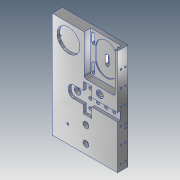
# Autodesk Inventor part: footbracket
Saved by Autodesk Inventor 2019 (Build 230136000, 136)
## iProperties
Created: 2019-01-05
Part Number: footbracket
Material: Aluminum 6061
Document SubType Name: Modeling
Designer: LillaHunden
Density: 2.7 g/cm^3
Appearance: Aluminum - Flat
Mass: 911.932 g
Surface Area: 667.083 cm^2
Volume: 337.752 cm^3
Author: LillaHunden
Autodesk Inventor part; units mm, degrees
ref_plane "YZ Plane" through (0, 0, 0) normal (1, 0, 0) x (0, 1, 0)
ref_plane "XZ Plane" through (0, 0, 0) normal (0, 1, 0) x (-1, 0, 0)
ref_plane "XY Plane" through (0, 0, 0) normal (0, 0, 1) x (1, 0, 0)
sketch "Sketch1" plane through (0, 0, 0) normal (0, 0, 1) x (1, 0, 0)
  line L0 (13.3, -8.75) -> (13.3, -10.75) construction
  line L1 (13.3, -10.75) -> (32.2, -10.75) construction
  line L2 (32.2, -10.75) -> (32.2, 3) construction
  line L3 (32.2, 3) -> (14.5, 3) construction
  line L4 (14.5, 3) -> (14.5, 0) construction
  line L5 (14.5, 0) -> (-0.1, 0) construction
  line L6 (-0.1, 0) -> (-0.1, 3) construction
  line L7 (-0.1, 3) -> (-17.8, 3) construction
  line L8 (-17.8, 3) -> (-17.8, -10.75) construction
  line L9 (-17.8, -10.75) -> (1.1, -10.75) construction
  line L10 (1.1, -10.75) -> (1.1, -8.75) construction
  line L11 (1.1, -8.75) -> (13.3, -8.75) construction
  line L12 (14.4, 0) -> (0, 0) construction
  line L13 (14.4, 0) -> (14.4, 50) construction
  line L14 (0, 50) -> (14.4, 50) construction
  line L15 (0, 0) -> (0, 50) construction
  line L16 (-60.1, -96.5) -> (59.9, -96.5)
  line L17 (59.9, -96.5) -> (59.9, 96.5)
  line L18 (59.9, 96.5) -> (-60.1, 96.5)
  line L19 (-60.1, 96.5) -> (-60.1, -96.5)
  point P0 (-60.1, 0)
  point P1 (-0.1, -96.5)
  dimension "d0" = 120
  dimension "d1" = 193
  constraints: 8 end point, 2 midpoint, 2 parallel, 1 horizontal, 1 horizontal alignment, 1 perpendicular, 1 vertical alignment
  measures "d0" distance of L18.end L17.end
  measures "d1" distance of L17.end L16.end
extrude "Extrusion1" add sketch "Sketch1" along normal mid plane 19
sketch "Sketch2" plane through (0, 0, 9.5) normal (0, 0, 1) x (1, 0, 0)
  circle A0 centre (-30.1, 68.5) radius 21
  line L0 (-60.1, 96.5) -> (-60.1, -96.5) projected
  line L1 (59.9, 96.5) -> (-60.1, 96.5) projected
  point P0 (0, 0)
  dimension "d4" = 42
  dimension "d5" = 30
  dimension "d6" = 28
  constraints: 1 centre point
  measures "d4" diameter of A0
  measures "d5" distance from line of L0 A0.centre
  measures "d6" distance from line of L1 A0.centre
extrude "Extrusion2" cut sketch "Sketch2" against normal blind 5
sketch "Sketch5" plane through (0, 0, 9.5) normal (0, 0, 1) x (1, 0, 0)
  circle A0 centre (-31.1, -64.5) radius 2
  line L0 (-60.1, -96.5) -> (59.9, -96.5) projected
  line L1 (-60.1, 96.5) -> (-60.1, -96.5) projected
  point P0 (0, 0)
  dimension "d20" = 4
  dimension "d21" = 32
  dimension "d22" = 29
  constraints: 1 centre point
  measures "d20" diameter of A0
  measures "d21" distance from line of L0 A0.centre
  measures "d22" distance from line of L1 A0.centre
extrude "Extrusion5" cut sketch "Sketch5" against normal through all
sketch "Sketch3" plane through (0, 0, 9.5) normal (0, 0, 1) x (1, 0, 0)
  circle A0 centre (1.9, -49.5) radius 5.5
  circle A1 centre (1.9, -79.5) radius 5.5
  line L0 (-60.1, 96.5) -> (-60.1, -96.5) projected
  line L1 (-60.1, -96.5) -> (59.9, -96.5) projected
  line L2 (1.9, -49.5) -> (1.9, -79.5) construction
  circle A2 centre (-31.1, -64.5) radius 2 projected
  line L3 (-31.1, -64.5) -> (-16.1488, -64.5) construction
  point P0 (0, 0)
  dimension "d9" = 11
  dimension "d10" = 11
  dimension "d11" = 62
  dimension "d25" = 47
  constraints: 4 end point, 2 centre point, 1 horizontal, 1 symmetric about line, 1 vertical, 1 vertical alignment
  measures "d9" diameter of A0
  measures "d10" diameter of A1
  measures "d11" distance from line of L0 L2.start
  measures "d25" distance from line of L1 L2.start
extrude "Extrusion3" cut sketch "Sketch3" against normal blind 7.14 contours A0 | A1
sketch "Sketch4" plane through (1.9, -49.5, 2.36) normal (0, 0, 1) x (1, 0, 0)
  circle A0 centre (0, -30) radius 5.5 projected
  circle A1 centre (0, 0) radius 5.5 projected
  circle A2 centre (0, 0) radius 3.465
  circle A3 centre (0, -30) radius 3.465
  point P0 (-1.9, 49.5)
  dimension "d16" = 6.93
  dimension "d17" = 6.93
  constraints: 2 centre point, 2 coincident
  measures "d16" diameter of A2
  measures "d17" diameter of A3
extrude "Extrusion4" cut sketch "Sketch4" against normal through all contours A2 | A3
sketch "Sketch6" plane through (0, 0, -9.5) normal (0, 0, -1) x (-1, 0, 0)
  circle A0 centre (31.1, -64.5) radius 2 projected
  circle A1 centre (31.1, -64.5) radius 21
  point P0 (0, 0)
  dimension "d26" = 42
  constraints: 1 centre point, 1 coincident
  measures "d26" diameter of A1
extrude "Extrusion6" cut sketch "Sketch6" against normal blind 5
sketch "Sketch7" plane through (0, 0, -9.5) normal (0, 0, -1) x (-1, 0, 0)
  line L0 (16.4, -52) -> (16.4, -96.5)
  line L1 (60.1, -96.5) -> (60.1, 96.5) projected
  line L2 (16.4, -52) -> (60.1, -52)
  line L3 (-59.9, -96.5) -> (60.1, -96.5) projected
  point P0 (0, 0)
  dimension "d29" = 43.7
  dimension "d30" = 44.5
  constraints: 4 end point, 2 point on line, 1 horizontal, 1 vertical
  measures "d29" distance between parallel lines of L1 L0
  measures "d30" distance between parallel lines of L3 L2
extrude "Extrusion7" cut sketch "Sketch7" against normal blind 3.3
sketch "Sketch8" plane through (0, 0, 9.5) normal (0, 0, 1) x (1, 0, 0)
  line L0 (8.9, -15.7) -> (58.9, -15.7) construction
  line L1 (58.9, -15.7) -> (58.9, -1.3) construction
  line L2 (8.9, -1.3) -> (58.9, -1.3) construction
  line L3 (-1.85, 16.5) -> (11.9, 16.5) construction
  line L4 (11.9, 16.5) -> (11.9, -1.2) construction
  line L5 (-1.85, -2.4) -> (-1.85, 16.5) construction
  line L6 (-7.85, -3) -> (-7.85, -14) construction
  line L7 (-1.85, -33.5) -> (-1.85, -14.6) construction
  line L8 (11.9, -33.5) -> (-1.85, -33.5) construction
  line L9 (11.9, -15.8) -> (11.9, -33.5) construction
  line L10 (-7.85, -3) -> (-7.85, -1) construction
  line L11 (-7.85, -1) -> (-1.85, -1) construction
  line L12 (-7.85, -14) -> (-7.85, -16) construction
  line L13 (-7.85, -16) -> (-1.85, -16) construction
  line L14 (59.9, -0.8) -> (59.9, -16.2)
  line L15 (59.9, -16.2) -> (12.4, -16.2)
  line L16 (12.4, -0.8) -> (12.4, -34)
  line L17 (12.4, -34) -> (-2.35, -34)
  line L18 (-2.35, -34) -> (-2.35, -16.5)
  line L19 (12.4, -16.2) -> (12.4, 17)
  line L20 (12.4, 17) -> (-2.35, 17)
  line L21 (-2.35, 17) -> (-2.35, -0.5)
  line L22 (-2.35, -0.5) -> (-8.35, -0.5)
  line L23 (-8.35, -0.5) -> (-8.35, -3)
  line L24 (-8.35, -3) -> (-8.35, -14)
  line L25 (-8.35, -14) -> (-8.35, -16.5)
  line L26 (-8.35, -16.5) -> (-2.35, -16.5)
  line L27 (12.4, -0.8) -> (59.9, -0.8)
  line L28 (12.4, -0.8) -> (59.9, -0.8)
  line L29 (59.9, -0.8) -> (59.9, -16.2)
  line L30 (59.9, -16.2) -> (12.4, -16.2)
  line L31 (12.4, -16.2) -> (12.4, -0.8)
  point P0 (0, 0)
  point P1 (59.9, -8.5)
  point P2 (59.9, 96.5)
  dimension "d33" = 2
  dimension "d34" = 2
  dimension "d36" = 0.5
  dimension "d38" = 0.5
  dimension "d44" = 0.5
  dimension "d45" = 0.5
  dimension "d46" = 0.5
  constraints: 44 end point, 5 point on line, 4 perpendicular, 2 parallel, 1 horizontal, 1 midpoint, 1 vertical, 1 vertical alignment, 2 other
  measures "d33" distance of L6.start L10.end
  measures "d34" distance of L6.end L12.end
  measures "d36" distance between parallel lines of L9 L16
  measures "d38" distance between parallel lines of L11 L22
  measures "d44" distance between parallel lines of L15 L0
  measures "d45" distance between parallel lines of L2 L27
  measures "d46" distance between parallel lines of L3 L20
extrude "Extrusion8" cut sketch "Sketch8" against normal blind 5 contours L16 L17 L18 L26 L25 L24 L23 L22 L21 L20 L19
sketch "Sketch9" plane through (0, 0, 9.5) normal (0, 0, 1) x (1, 0, 0)
  line L0 (-12.85, 11.5) -> (-12.85, -28.5) construction
  line L1 (-12.85, -28.5) -> (-20.85, -28.5) construction
  line L2 (-20.85, 11.5) -> (-20.85, -28.5) construction
  line L3 (-12.85, 11.5) -> (-20.85, 11.5) construction
  line L4 (-12.85, -8.5) -> (-20.85, -8.5) construction
  circle A0 centre (-18.35, -8.5) radius 6.1
  line L5 (-8.35, -16.5) -> (-8.35, -0.5) projected
  point P0 (0, 0)
  dimension "d41" = 12.2
  dimension "d116" = 10
  constraints: 2 end point, 2 midpoint, 1 centre point, 1 perpendicular, 1 point on line
  measures "d41" diameter of A0
  measures "d116" distance from line of A0.centre L5
extrude "Extrusion9" cut sketch "Sketch9" against normal through all
sketch "Sketch10" plane through (0, 0, 9.5) normal (0, 0, 1) x (1, 0, 0)
  line L0 (8.9, -15.7) -> (58.9, -15.7) construction
  line L1 (8.9, -1.3) -> (58.9, -1.3) construction
  line L2 (12.4, 17) -> (12.4, -34) construction
  line L3 (12.4, 17) -> (12.4, -34) projected
  line L4 (59.9, 96.5) -> (59.9, -96.5) projected
  line L5 (59.9, -1) -> (59.9, -16)
  line L6 (59.9, -16) -> (12.4, -16)
  line L7 (12.4, -16) -> (12.4, -1.3)
  line L8 (8.9, -1) -> (59.9, -1)
  line L9 (59.9, -96.5) -> (59.9, 96.5) projected
  line L10 (12.4, -1.3) -> (12.4, -1)
  point P0 (0, 0)
  dimension "d49" = 0.3
  dimension "d50" = 0.3
  constraints: 10 end point, 6 point on line, 2 parallel
  measures "d49" distance between parallel lines of L0 L6
  measures "d50" distance between parallel lines of L1 L8
extrude "Extrusion10" cut sketch "Sketch10" against normal up to surface (5 mm away)
sketch "Sketch12" plane through (0, 0, 9.5) normal (0, 0, 1) x (1, 0, 0)
  line L0 (55.1541, 83.9537) -> (55.1541, 33.9537) construction
  arc A0 (52.1541, 30.9537) -> (55.1541, 33.9537) centre (52.1541, 33.9537) ccw construction
  line L1 (52.1541, 30.9537) -> (2.1541, 30.9537) construction
  arc A1 (55.1541, 83.9537) -> (52.1541, 86.9537) centre (52.1541, 83.9537) ccw construction
  line L2 (2.1541, 86.9537) -> (52.1541, 86.9537) construction
  arc A2 (2.1541, 86.9537) -> (-0.8459, 83.9537) centre (2.1541, 83.9537) ccw construction
  line L3 (-0.8459, 33.9537) -> (-0.8459, 83.9537) construction
  arc A3 (-0.8459, 33.9537) -> (2.1541, 30.9537) centre (2.1541, 33.9537) ccw construction
  line L4 (-1.3459, 22.9537) -> (55.6541, 22.9537)
  line L5 (55.6541, 22.9537) -> (55.6541, 96.9537)
  line L6 (55.6541, 96.9537) -> (-1.3459, 96.9537)
  line L7 (-1.3459, 96.9537) -> (-1.3459, 22.9537)
  point P0 (0, 0)
  dimension "d54" = 8
  dimension "d55" = 0.5
  dimension "d56" = 0.5
  dimension "d57" = 10
  constraints: 8 end point, 2 parallel, 1 horizontal, 1 perpendicular, 1 other
  measures "d54" distance between parallel lines of L4 L1
  measures "d55" distance between parallel lines of L3 L7
  measures "d56" distance between parallel lines of L5 L0
  measures "d57" distance between parallel lines of L2 L6
extrude "Extrusion12" cut sketch "Sketch12" against normal blind 12
sketch "Sketch13" plane through (0, 0, -2.5) normal (0, 0, 1) x (1, 0, 0)
  circle A0 centre (50.7241, 27.8837) radius 2.6 construction
  circle A1 centre (50.7241, 75.0237) radius 2.6 construction
  circle A2 centre (3.5841, 75.0237) radius 2.6 construction
  circle A3 centre (3.5841, 27.8837) radius 2.6 construction
  line L0 (3.5841, 25.2837) -> (3.5841, 45.2837) construction
  line L1 (0.9841, 27.8837) -> (0.9841, 42.6837)
  line L2 (6.1841, 42.6837) -> (6.1841, 27.8837)
  arc A4 (0.9841, 27.8837) -> (6.1841, 27.8837) centre (3.5841, 27.8837) ccw
  arc A5 (6.1841, 42.6837) -> (0.9841, 42.6837) centre (3.5841, 42.6837) ccw
  line L3 (3.5841, 72.4237) -> (3.5841, 92.4237) construction
  line L4 (0.9841, 75.0237) -> (0.9841, 89.8237)
  line L5 (6.1841, 89.8237) -> (6.1841, 75.0237)
  arc A6 (0.9841, 75.0237) -> (6.1841, 75.0237) centre (3.5841, 75.0237) ccw
  arc A7 (6.1841, 89.8237) -> (0.9841, 89.8237) centre (3.5841, 89.8237) ccw
  line L6 (50.7241, 72.4237) -> (50.7241, 92.4237) construction
  line L7 (48.1241, 75.0237) -> (48.1241, 89.8237)
  line L8 (53.3241, 89.8237) -> (53.3241, 75.0237)
  arc A8 (48.1241, 75.0237) -> (53.3241, 75.0237) centre (50.7241, 75.0237) ccw
  arc A9 (53.3241, 89.8237) -> (48.1241, 89.8237) centre (50.7241, 89.8237) ccw
  line L9 (50.7241, 25.2837) -> (50.7241, 45.2837) construction
  line L10 (48.1241, 27.8837) -> (48.1241, 42.6837)
  line L11 (53.3241, 42.6837) -> (53.3241, 27.8837)
  arc A10 (48.1241, 27.8837) -> (53.3241, 27.8837) centre (50.7241, 27.8837) ccw
  arc A11 (53.3241, 42.6837) -> (48.1241, 42.6837) centre (50.7241, 42.6837) ccw
  point P0 (0, 0)
  point P1 (3.5841, 35.2837)
  point P2 (3.5841, 82.4237)
  point P3 (50.7241, 82.4237)
  point P4 (50.7241, 35.2837)
  dimension "d60" = 20
  dimension "d61" = 20
  dimension "d62" = 20
  dimension "d63" = 20
  dimension "d117" = 5.2
  dimension "d118" = 5.2
  constraints: 32 end point, 24 point on circle, 16 tangent, 12 point on line, 8 centre point, 5 parallel, 4 midpoint, 4 vertical alignment, 1 vertical, 4 other
  measures "d60" distance of L0.start L0.end
  measures "d61" distance of L3.start L3.end
  measures "d62" distance of L6.start L6.end
  measures "d63" distance of L9.start L9.end
  measures "d117" distance between parallel lines of L5 L4
  measures "d118" distance between parallel lines of L1 L2
extrude "Extrusion13" cut sketch "Sketch13" against normal through all
sketch "Sketch14" plane through (0, 0, -2.5) normal (0, 0, 1) x (1, 0, 0)
  circle A0 centre (27.1541, 51.4537) radius 19.5 construction
  arc A1 (7.6604, 46.9821) -> (46.6279, 46.8964) centre (27.1541, 51.4537) ccw
  line L0 (46.6279, 72.4633) -> (46.6279, 46.8964)
  line L1 (7.6604, 46.9821) -> (7.6604, 70.9586)
  arc A2 (46.6279, 70.4442) -> (7.6604, 70.9586) centre (27.1541, 71.4537) ccw
  point P0 (0, 0)
  point P1 (46.6279, 67.5038)
  point P2 (27.1541, 90.9537)
  dimension "d67" = 39
  dimension "d68" = 0.5
  dimension "d120" = 39
  dimension "d121" = 20
  constraints: 5 point on circle, 4 end point, 2 centre point, 2 point on line, 2 vertical, 2 vertical alignment
  measures "d67" diameter of A0
  measures "d68" radial gap between concentric circles of A0 A1
  measures "d120" diameter of A2
  measures "d121" distance of A0.centre A2.centre
extrude "Extrusion14" cut sketch "Sketch14" against normal blind 1.85 contours L1 A2 L0 A1
sketch "Sketch15" plane through (0, 0, -4.35) normal (0, 0, 1) x (1, 0, 0)
  circle A0 centre (27.1541, 51.4537) radius 3.18 construction
  line L0 (27.1541, 48.2737) -> (27.1541, 68.2737) construction
  line L1 (30.4041, 51.5237) -> (30.4041, 65.0237)
  line L2 (23.9041, 65.0237) -> (23.9041, 51.5237)
  arc A1 (23.9041, 51.5237) -> (30.4041, 51.5237) centre (27.1541, 51.5237) ccw
  arc A2 (30.4041, 65.0237) -> (23.9041, 65.0237) centre (27.1541, 65.0237) ccw
  point P0 (0, 0)
  point P1 (27.1541, 58.2737)
  dimension "d72" = 20
  dimension "d73" = 6.5
  constraints: 8 end point, 6 point on circle, 4 tangent, 2 centre point, 2 point on line, 1 midpoint, 1 parallel, 1 vertical, 1 vertical alignment, 1 other
  measures "d72" distance of L0.start L0.end
  measures "d73" diameter of A2
extrude "Extrusion15" cut sketch "Sketch15" against normal through all
sketch "Sketch16" plane through (0, 0, 9.5) normal (0, 0, 1) x (1, 0, 0)
  circle A0 centre (27.1817, 11.6) radius 4.7625 projected
  point P0 (0, 0)
extrude "Extrusion16" cut sketch "Sketch16" against normal through all
sketch "Sketch17" plane through (0, 0, -9.5) normal (0, 0, -1) x (-1, 0, 0)
  circle A0 centre (-48.9, -8.5) radius 2.067 construction
  circle A1 centre (-33.9, -8.5) radius 2.067 construction
  circle A2 centre (-18.9, -8.5) radius 2.067 construction
  circle A3 centre (-5.025, -24.65) radius 2.067 construction
  circle A4 centre (-5.025, -8.5) radius 2.067 construction
  circle A5 centre (-5.025, 7.65) radius 2.067 construction
  circle A6 centre (-5.025, -24.65) radius 3
  circle A7 centre (-5.025, -8.5) radius 3
  circle A8 centre (-18.9, -8.5) radius 3
  circle A9 centre (-33.9, -8.5) radius 3
  circle A10 centre (-48.9, -8.5) radius 3
  circle A11 centre (-5.025, 7.65) radius 3
  point P0 (0, 0)
  dimension "d78" = 6
  dimension "d79" = 6
  dimension "d80" = 6
  dimension "d81" = 6
  dimension "d82" = 6
  dimension "d83" = 6
  constraints: 6 centre point
  measures "d78" diameter of A7
  measures "d79" diameter of A6
  measures "d80" diameter of A11
  measures "d81" diameter of A8
  measures "d82" diameter of A9
  measures "d83" diameter of A10
extrude "Extrusion17" cut sketch "Sketch17" against normal through all
sketch "Sketch18" plane through (0, 0, -9.5) normal (0, 0, -1) x (-1, 0, 0)
  line L0 (-59.9, -1) -> (-12.4, -1) projected
  line L1 (-56.4, -8.5) -> (2.475, -8.5) construction
  line L2 (-48.9, -16) -> (-5.025, -16)
  line L3 (-5.025, -1) -> (-48.9, -1)
  arc A0 (-48.9, -1) -> (-48.9, -16) centre (-48.9, -8.5) ccw
  arc A1 (-5.025, -16) -> (-5.025, -1) centre (-5.025, -8.5) ccw
  line L4 (-5.025, -32.15) -> (-5.025, 13.5608) construction
  line L5 (-12.525, -24.65) -> (-12.525, 6.0608)
  line L6 (2.475, 6.0608) -> (2.475, -24.65)
  arc A2 (-12.525, -24.65) -> (2.475, -24.65) centre (-5.025, -24.65) ccw
  arc A3 (2.475, 6.0608) -> (-12.525, 6.0608) centre (-5.025, 6.0608) ccw
  point P0 (-5.025, 7.65)
  point P1 (-26.9625, -8.5)
  point P2 (-5.025, -9.2946)
  dimension "d94" = 7.5
  dimension "d95" = 7.5
  constraints: 16 end point, 12 point on circle, 8 tangent, 6 point on line, 4 centre point, 3 coincident, 2 midpoint, 2 parallel, 1 horizontal, 1 perpendicular
  measures "d94" radius of A2
  measures "d95" radius of A1
extrude "Extrusion18" cut sketch "Sketch18" against normal blind 7
sketch "Sketch19" plane through (0, 0, -9.5) normal (0, 0, -1) x (-1, 0, 0)
  circle A0 centre (18.35, -8.5) radius 6.1 projected
  circle A1 centre (18.35, -8.5) radius 11.7114
  point P0 (0, 0)
  constraints: 1 centre point, 1 coincident
extrude "Extrusion19" cut sketch "Sketch19" against normal up to surface (7 mm away)
fillet "Fillet1" radius 4 2 edges at (55.6541, 22.9537, 3.5) (-1.3459, 22.9537, 3.5)
sketch "Sketch20" plane through (0, 0, 9.5) normal (0, 0, 1) x (1, 0, 0)
  circle A0 centre (-18.35, -8.5) radius 6.1 projected
  arc A1 (-18.35, -0.5) -> (-18.35, -16.5) centre (-18.35, -8.5) ccw
  line L0 (-8.35, -0.5) -> (-2.35, -0.5) projected
  line L1 (-2.35, -16.5) -> (-8.35, -16.5) projected
  line L2 (-8.35, -16.5) -> (-18.35, -16.5)
  line L3 (-8.35, -0.5) -> (-18.35, -0.5)
  line L4 (-8.35, -16.5) -> (-8.35, -0.5) projected
  line L5 (-2.35, -0.5) -> (-2.35, 17) projected
  line L6 (-29.85, -19.5) -> (-2.35, -19.5)
  line L7 (-2.35, -19.5) -> (-2.35, 2.5)
  line L8 (-2.35, 2.5) -> (-29.85, 2.5)
  line L9 (-29.85, 2.5) -> (-29.85, -19.5)
  point P0 (0, 0)
  dimension "d112" = 3
  dimension "d113" = 3
  dimension "d114" = 11.5
  constraints: 12 end point, 3 parallel, 2 point on circle, 1 centre point, 1 coincident, 1 collinear, 1 horizontal, 1 perpendicular, 1 point on line, 1 tangent
  measures "d112" distance between parallel lines of L6 L1
  measures "d113" distance between parallel lines of L0 L8
  measures "d114" distance from line of L9 A1.centre
extrude "Extrusion20" cut sketch "Sketch20" against normal up to surface (5 mm away)
sketch "Sketch21" plane through (0, 0, 9.5) normal (0, 0, 1) x (1, 0, 0)
  circle A0 centre (-0.9358, -32.5858) radius 2
  line L0 (12.4, -34) -> (-2.35, -34) projected
  line L1 (-2.35, -34) -> (3.6865, -27.9635) construction
  line L2 (12.4, -16) -> (12.4, -34) projected
  line L3 (12.4, -34) -> (9.5716, -31.1716) construction
  line L4 (-2.35, 2.5) -> (-2.35, 17) projected
  line L5 (-2.35, 17) -> (2.4494, 12.2006) construction
  line L6 (12.4, 17) -> (9.5716, 14.1716) construction
  line L7 (12.4, 17) -> (12.4, -1) projected
  circle A1 centre (10.9858, -32.5858) radius 2
  circle A2 centre (-0.9358, 15.5858) radius 2
  circle A3 centre (10.9858, 15.5858) radius 2
  point P0 (0, 0)
  point P1 (-2.35, -0.5)
  dimension "d102" = 4
  dimension "d107" = 4
  dimension "d108" = 4
  dimension "d109" = 4
  dimension "d103" = 45
  dimension "d104" = 45
  dimension "d105" = 45
  dimension "d106" = 45
  constraints: 8 end point, 2 midpoint, 2 point on line, 12 other
  measures "d103" angle of L0 L1
  measures "d104" angle of L4 L5
  measures "d105" angle of L7 L6
  measures "d106" angle of L0 L3
extrude "Extrusion21" cut sketch "Sketch21" against normal up to surface (5 mm away)
fillet "Fillet2" radius 8 2 edges at (-29.85, -19.5, 7) (-29.85, 2.5, 7)
sketch "Sketch22" plane through (0, 0, 9.5) normal (0, 0, 1) x (1, 0, 0)
  circle A0 centre (27.1817, 11.6) radius 4.7625 projected
  circle A1 centre (27.1817, 11.6) radius 6.5
  point P0 (0, 0)
  dimension "d122" = 13
  constraints: 1 centre point, 1 coincident
  measures "d122" diameter of A1
extrude "Extrusion22" cut sketch "Sketch22" against normal blind 2 contours A0 | A1
sketch "Sketch23" plane through (0, 0, -9.5) normal (0, 0, -1) x (-1, 0, 0)
  circle A0 centre (-27.1817, 11.6) radius 6.5 projected
  point P0 (0, 0)
extrude "Extrusion23" cut sketch "Sketch23" against normal blind 2
sketch "Sketch24" plane through (-60.1, -96.5, 9.5) normal (-1, 0, 0) x (0, 0, 1)
  circle A0 centre (-6.3333, 160.8333) radius 2.25 construction
  circle A1 centre (-14.3333, 160.8333) radius 2.25 construction
  circle A2 centre (-14.3333, 128.6667) radius 2.25 construction
  circle A3 centre (-6.3333, 128.6667) radius 2.25 construction
  circle A4 centre (-6.3333, 96.5) radius 2.25 construction
  circle A5 centre (-14.3333, 96.5) radius 2.25 construction
  circle A6 centre (-14.3333, 64.3333) radius 2.25 construction
  circle A7 centre (-6.3333, 64.3333) radius 2.25 construction
  circle A8 centre (-6.3333, 32.1667) radius 2.25 construction
  circle A9 centre (-14.3333, 32.1667) radius 2.25 construction
  point P0 (-9.5, 96.5)
  constraints: 1 centre point
hole "Hole1" at (-60.1, 64.3333, -4.8333) at (-60.1, 64.3333, 3.1667) at (-60.1, 32.1667, 3.1667) at (-60.1, 32.1667, -4.8333) at (-60.1, 0, -4.8333) at (-60.1, 0, 3.1667) at (-60.1, -32.1667, 3.1667) at (-60.1, -32.1667, -4.8333) at (-60.1, -64.3333, 3.1667) direction (1, 0, 0) diameter 3.242 depth 11.8 thread size "M4x0.7" class "6H" standard "ISO Metric profile"
sketch "Sketch25" plane through (59.9, -96.5, -9.5) normal (1, 0, 0) x (0, 0, -1)
  circle A0 centre (-4.6667, 64.3333) radius 1.621 construction
  circle A1 centre (-12.6667, 96.5) radius 1.621 construction
  circle A2 centre (-4.6667, 128.6667) radius 1.621 construction
  circle A3 centre (-12.6667, 160.8333) radius 1.621 construction
  circle A4 centre (-4.6667, 160.8333) radius 1.621 construction
  circle A5 centre (-12.6667, 128.6667) radius 1.621 construction
  circle A6 centre (-4.6667, 96.5) radius 1.621 construction
  circle A7 centre (-12.6667, 64.3333) radius 1.621 construction
  circle A8 centre (-12.6667, 32.1667) radius 1.621 construction
  line L0 (0, 44.5) -> (-3.3, 44.5) construction
  line L1 (-3.3, 44.5) -> (-3.3, 0) construction
  line L2 (-19, 0) -> (-3.3, 0) construction
  line L3 (-19, 193) -> (-19, 0) construction
  line L4 (0, 193) -> (-19, 193) construction
  line L5 (0, 44.5) -> (0, 193) construction
  circle A9 centre (-4.6667, 10.8333) radius 3.25 projected
  circle A10 centre (-4.6667, 40.8333) radius 3.25 projected
  circle A11 centre (-12.6667, 70.8333) radius 3.25 projected
  circle A12 centre (-4.6667, 100.8333) radius 3.25 projected
  circle A13 centre (-4.6667, 130.8333) radius 3.25 projected
  circle A14 centre (-12.6667, 160.8333) radius 3.25 projected
  circle A15 centre (-4.6667, 160.8333) radius 3.25 projected
  circle A16 centre (-12.6667, 130.8333) radius 3.25 projected
  circle A17 centre (-12.6667, 100.8333) radius 3.25 projected
  circle A18 centre (-4.6667, 70.8333) radius 3.25 projected
  circle A19 centre (-12.6667, 40.8333) radius 3.25 projected
  circle A20 centre (-12.6667, 10.8333) radius 3.25 projected
  circle A21 centre (-22.7521, 16) radius 3.25 projected
  circle A22 centre (-22.7521, -174) radius 3.25 projected
  circle A23 centre (-22.7521, -157) radius 3.25 projected
  circle A24 centre (-22.7521, 33) radius 3.25 projected
  line L6 (4, -32.5) -> (20, -32.5) projected
  arc A25 (20, -39.5) -> (20, -32.5) centre (20, -36) ccw projected
  line L7 (20, -39.5) -> (4, -39.5) projected
  arc A26 (4, -32.5) -> (4, -39.5) centre (4, -36) ccw projected
  arc A27 (43.57, -15.03) -> (43.57, -9.83) centre (43.57, -12.43) ccw projected
  line L8 (43.57, -15.03) -> (27.57, -15.03) projected
  arc A28 (27.57, -9.83) -> (27.57, -15.03) centre (27.57, -12.43) ccw projected
  line L9 (27.57, -9.83) -> (43.57, -9.83) projected
  arc A29 (-3.57, -15.03) -> (-3.57, -9.83) centre (-3.57, -12.43) ccw projected
  line L10 (-3.57, -15.03) -> (-19.57, -15.03) projected
  arc A30 (-19.57, -9.83) -> (-19.57, -15.03) centre (-19.57, -12.43) ccw projected
  line L11 (-19.57, -9.83) -> (-3.57, -9.83) projected
  arc A31 (-3.57, -62.17) -> (-3.57, -56.97) centre (-3.57, -59.57) ccw projected
  line L12 (-3.57, -62.17) -> (-19.57, -62.17) projected
  arc A32 (-19.57, -56.97) -> (-19.57, -62.17) centre (-19.57, -59.57) ccw projected
  line L13 (-19.57, -56.97) -> (-3.57, -56.97) projected
  arc A33 (43.57, -62.17) -> (43.57, -56.97) centre (43.57, -59.57) ccw projected
  line L14 (43.57, -62.17) -> (27.57, -62.17) projected
  arc A34 (27.57, -56.97) -> (27.57, -62.17) centre (27.57, -59.57) ccw projected
  line L15 (27.57, -56.97) -> (43.57, -56.97) projected
  arc A35 (-26.9823, 31) -> (-28.9823, 33.8284) centre (-29.9823, 31) ccw projected
  line L16 (-26.9823, 31) -> (-26.9823, 18) projected
  arc A36 (-28.9823, 15.1716) -> (-26.9823, 18) centre (-29.9823, 18) ccw projected
  line L17 (-28.9823, 15.1716) -> (-28.9823, -156.1716) projected
  arc A37 (-26.9823, -159) -> (-28.9823, -156.1716) centre (-29.9823, -159) ccw projected
  line L18 (-26.9823, -159) -> (-26.9823, -172) projected
  arc A38 (-28.9823, -174.8284) -> (-26.9823, -172) centre (-29.9823, -172) ccw projected
  line L19 (-28.9823, -174.8284) -> (-28.9823, -178) projected
  line L20 (-28.9823, -178) -> (48, -178) projected
  line L21 (48, -178) -> (48, 193) projected
  line L22 (48, 193) -> (-28.9823, 193) projected
  line L23 (-28.9823, 193) -> (-28.9823, 33.8284) projected
  circle A39 centre (-15.9823, -84.3) radius 5.2625 projected
  point P0 (-3.9778, 64.4692)
  constraints: 12 coincident
hole "Hole2" at (59.9, -32.1667, -4.8333) at (59.9, 64.3333, 3.1667) at (59.9, 64.3333, -4.8333) at (59.9, 34.3333, -4.8333) at (59.9, 34.3333, 3.1667) at (59.9, 4.3333, 3.1667) at (59.9, 4.3333, -4.8333) at (59.9, -25.6667, -4.8333) at (59.9, -25.6667, 3.1667) at (59.9, -55.6667, -4.8333) at (59.9, -55.6667, 3.1667) at (59.9, -85.6667, 3.1667) at (59.9, -85.6667, -4.8333) direction (-1, 0, 0) diameter 3.242 depth 11.8 thread size "M4x0.7" class "6H" standard "ISO Metric profile"
equation "\"d34\" = d33"
equation "\"d61\" = d60"
equation "\"d62\" = d60"
equation "\"d63\" = d60"
equation "\"d117\" = d118"
equation "\"d120\" = d67"
equation "\"d78\" = d79"
equation "\"d80\" = d78"
equation "\"d81\" = d78"
equation "\"d82\" = d79"
equation "\"d83\" = d79"
equation "\"d95\" = d94"
equation "\"d113\" = d112"
equation "\"d102\" = d107"
equation "\"d108\" = d102"
equation "\"d109\" = d107"
body "Solid1"
